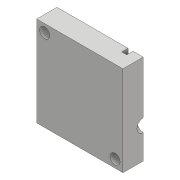
# Autodesk Inventor part: knee_motor_hemi
Saved by Autodesk Inventor 2017 (Build 210142000, 142)
## iProperties
Created: 2019-03-28
Part Number: knee_motor_hemi
Material: Generic
Document SubType Name: Modeling
Designer: mfans
Density: 1 g/cm^3
Appearance: Default
Author: mfans
Autodesk Inventor part; units mm, degrees
ref_plane "YZ Plane" through (0, 0, 0) normal (1, 0, 0) x (0, 1, 0)
ref_plane "XZ Plane" through (0, 0, 0) normal (0, 1, 0) x (-1, 0, 0)
ref_plane "XY Plane" through (0, 0, 0) normal (0, 0, 1) x (1, 0, 0)
sketch "Sketch1" plane through (0, 0, 0) normal (0, 1, 0) x (-1, 0, 0)
  line L0 (16, 17.75) -> (-16, 17.75)
  line L1 (-16, 17.75) -> (-16, -17.75)
  line L2 (-16, -17.75) -> (16, -17.75)
  line L3 (16, -17.75) -> (16, 17.75)
  line L4 (16, 17.75) -> (-16, -17.75) construction
  line L5 (-16, 17.75) -> (16, -17.75) construction
  point P0 (0, 0)
  dimension "d0" = 32
  dimension "d1" = 35.5
  constraints: 12 end point, 2 midpoint, 2 parallel, 1 horizontal, 1 perpendicular
  measures "d0" distance of L2.end L1.end
  measures "d1" distance of L0.end L1.end
extrude "Extrusion1" add sketch "Sketch1" along normal blind 8
sketch "Sketch2" plane through (0, 8, 0) normal (0, 1, 0) x (1, 0, 0)
  line L0 (-11, 11.5) -> (14, 11.5)
  line L1 (14, 11.5) -> (14, -11.5)
  line L2 (14, -11.5) -> (-11, -11.5)
  line L3 (-11, -11.5) -> (-11, 11.5)
  line L4 (-11, 11.5) -> (14, -11.5) construction
  line L5 (14, 11.5) -> (-11, -11.5) construction
  line L6 (16, -17.75) -> (16, 17.75) projected
  point P0 (0, 0)
  point P1 (1.5, 0)
  dimension "d4" = 0
  dimension "d5" = 2
  dimension "d6" = 25
  dimension "d13" = 23
  constraints: 12 end point, 2 midpoint, 2 parallel, 1 horizontal, 1 perpendicular
  measures "d4" vertical distance of point (0, 0) point (1.5, 0)
  measures "d5" distance between parallel lines of L6 L1
  measures "d6" distance of L0.start L0.end
  measures "d13" distance of L0.end L1.end
extrude "Extrusion2" cut sketch "Sketch2" against normal blind 6
sketch "Sketch3" plane through (0, 8, 0) normal (0, 1, 0) x (1, 0, 0)
  line L0 (-7, -15.75) -> (-9.5, -15.75)
  line L1 (-9.5, -15.75) -> (-9.5, 15.75)
  line L2 (-9.5, 15.75) -> (-7, 15.75)
  line L3 (-7, 15.75) -> (-7, -15.75)
  line L4 (-7, -15.75) -> (-9.5, 15.75) construction
  line L5 (-9.5, -15.75) -> (-7, 15.75) construction
  line L6 (14, 11.5) -> (14, -11.5) projected
  point P0 (0, 0)
  point P1 (-8.25, 0)
  dimension "d9" = 21
  dimension "d10" = 2.5
  dimension "d11" = 0
  dimension "d12" = 31.5
  constraints: 12 end point, 2 midpoint, 2 parallel, 1 horizontal, 1 perpendicular
  measures "d9" distance between parallel lines of L6 L3
  measures "d10" distance between parallel lines of L1 L3
  measures "d11" vertical distance of point (0, 0) point (-8.25, 0)
  measures "d12" distance of L2.end L0.start
extrude "Extrusion3" cut sketch "Sketch3" against normal blind 6
sketch "Sketch4" plane through (-16, 0, -17.75) normal (-1, 0, 0) x (0, 0, 1)
  line L0 (6.25, 8) -> (6.25, 2) projected
  line L1 (6.25, 8) -> (29.25, 8) projected
  line L2 (6.25, 2) -> (29.25, 2) projected
  line L3 (18.25, 5) -> (17.4462, 5)
  line L4 (18.25, 11) -> (17.4462, 11)
  arc A0 (18.25, 5) -> (18.25, 11) centre (18.25, 8) ccw
  arc A1 (17.4462, 11) -> (17.4462, 5) centre (12.25, 8) ccw
  arc A2 (18.25, 8) -> (17.5, 10.9047) centre (12.25, 8) ccw
  point P0 (17.75, 0)
  dimension "d17" = 6
  constraints: 7 point on circle, 4 end point, 3 centre point, 2 point on line, 1 horizontal, 1 parallel, 1 tangent
  measures "d17" distance of A0.centre A1.centre
extrude "Extrusion4" cut sketch "Sketch4" against normal up to surface (30 mm away) contours A1 L4 A0 L1 | L1 A0 L3 A1
thicken "Thicken1" operation add thickness 2 both sides no extend neighbours yes toward (1, 0, 0) faces at (16, 5.3333, 5.9167)
sketch "Sketch6" plane through (18, 0, 17.75) normal (1, 0, 0) x (0, 0, -1)
  arc A0 (18.0538, 5) -> (29.25, 8) centre (23.25, 8) ccw projected
  circle A1 centre (23.25, 8) radius 2.5
  point P0 (17.75, 0)
  dimension "d26" = 5
  constraints: 1 centre point, 1 coincident
  measures "d26" diameter of A1
extrude "Extrusion6" cut sketch "Sketch6" against normal blind 2.5
fillet "Fillet2" radius 2.5 1 edges at (15.5, 5.5, -5.5)
sketch "Sketch7" plane through (0, 8, 0) normal (0, 1, 0) x (1, 0, 0)
  arc A0 (18, 8) -> (18, 3) centre (18, 5.5) ccw projected
  line L0 (18, 8) -> (18, 17.75) projected
  line L1 (18, 17.75) -> (-16, 17.75) projected
  line L2 (-16, 17.75) -> (-16, 11.5) projected
  line L3 (-16, 11.5) -> (-11, 11.5) projected
  line L4 (-11, 11.5) -> (-9.5, 11.5) projected
  line L5 (-9.5, 11.5) -> (-9.5, 15.75) projected
  line L6 (-9.5, 15.75) -> (-7, 15.75) projected
  line L7 (-7, 15.75) -> (-7, 11.5) projected
  line L8 (-7, 11.5) -> (14, 11.5) projected
  line L9 (14, 11.5) -> (14, -11.5) projected
  line L10 (14, -11.5) -> (-7, -11.5) projected
  line L11 (-7, -11.5) -> (-7, -15.75) projected
  line L12 (-7, -15.75) -> (-9.5, -15.75) projected
  line L13 (-9.5, -15.75) -> (-9.5, -11.5) projected
  line L14 (-9.5, -11.5) -> (-11, -11.5) projected
  line L15 (-11, -11.5) -> (-11, -3.5) projected
  line L16 (-11, -3.5) -> (-16, -3.5) projected
  line L17 (-16, -3.5) -> (-16, -17.75) projected
  line L18 (-16, -17.75) -> (18, -17.75) projected
  line L19 (18, -17.75) -> (18, 3) projected
  line L20 (-16, -17.75) -> (18, -17.75) projected
  line L21 (14, -11.5) -> (12, -11.5)
  line L22 (12, -11.5) -> (12, -17.75)
  line L23 (12, -17.75) -> (14, -17.75)
  line L24 (14, -17.75) -> (14, -11.5)
  point P0 (0, 0)
  dimension "d30" = 2
  constraints: 8 end point, 2 parallel, 1 horizontal, 1 perpendicular, 1 point on line
  measures "d30" distance of L23.end L22.end
extrude "Extrusion7" cut sketch "Sketch7" against normal blind 2.5 contours L18 L22 L10 L24
sketch "Sketch8" plane through (0, 8, 0) normal (0, 1, 0) x (1, 0, 0)
  line L0 (18, 17.75) -> (-16, 17.75) projected
  line L1 (18, 8) -> (18, 17.75) projected
  line L2 (-16, -17.75) -> (12, -17.75) projected
  line L3 (-16, -3.5) -> (-16, -17.75) projected
  point P0 (0, 0)
  point P1 (14.875, 14.625)
  point P2 (-12.875, -14.625)
  dimension "d33" = 3.125
  dimension "d34" = 3.125
  dimension "d35" = 3.125
  dimension "d36" = 3.125
  measures "d33" distance from line of L0 point (14.875, 14.625)
  measures "d34" distance from line of L1 point (14.875, 14.625)
  measures "d35" distance from line of L2 point (-12.875, -14.625)
  measures "d36" distance from line of L3 point (-12.875, -14.625)
hole "Hole1" at (14.875, 8, -14.625) at (-12.875, 8, 14.625) direction (0, -1, 0) diameter 4 end through all
body "Solid1"
